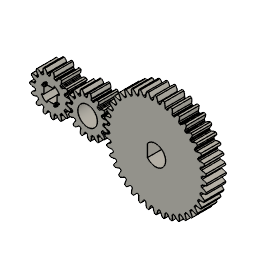
Dribbler Gears (Autodesk Fusion 360 design; units mm, degrees)
description: Spur Gear; Module: 1.5; Num Teeth: 18; Pressure Angle: 20.0; Backlash: 0.00 mm
part number: 2026-04-08-17-27-07-443
Autodesk Fusion 360 part; units mm, degrees
(part 1 of 6)
sketch "Base Circle" plane through (0, 0, 0) normal (0, 0, 1) x (1, 0, 0)
  circle A0 centre (0, 0) radius 9.4215
  circle A1 centre (0, 0) radius 2
extrude "Extrude12" add sketch "Base Circle" along normal blind 4 makes body 1
sketch "Gear Tooth" plane through (0, 0, 0) normal (0, 0, 1) x (1, 0, 0)
  spline S0 degree 5 poles (9.3831, -0.5088) (9.3863, -0.5089) (9.3927, -0.5089) (9.4023, -0.5088) (9.415, -0.5086) (9.431, -0.5081) (9.4469, -0.5073) (9.4629, -0.5063) (9.4789, -0.505) (9.4949, -0.5035) (9.5109, -0.5018) (9.5269, -0.4999) (9.5428, -0.4978) (9.5588, -0.4956) (9.5749, -0.4933) (9.5909, -0.4909) (9.6069, -0.4883) (9.6229, -0.4856) (9.6389, -0.4827) (9.6549, -0.4797) (9.6709, -0.4766) (9.6869, -0.4734) (9.7029, -0.4701) (9.7189, -0.4667) (9.7349, -0.4631) (9.7509, -0.4595) (9.7669, -0.4557) (9.7829, -0.4519) (9.7989, -0.4479) (9.8149, -0.4439) (9.8309, -0.4397) (9.8469, -0.4355) (9.8629, -0.4311) (9.8788, -0.4267) (9.8948, -0.4222) (9.9108, -0.4176) (9.9268, -0.4129) (9.9428, -0.4081) (9.9587, -0.4032) (9.9747, -0.3982) (9.9906, -0.3931) (10.0066, -0.388) (10.0225, -0.3828) (10.0385, -0.3775) (10.0544, -0.3721) (10.0704, -0.3666) (10.0863, -0.3611) (10.1022, -0.3554) (10.1181, -0.3497) (10.1341, -0.3439) (10.15, -0.338) (10.1659, -0.3321) (10.1818, -0.3261) (10.1977, -0.32) (10.2136, -0.3138) (10.2294, -0.3075) (10.2453, -0.3012) (10.2612, -0.2948) (10.277, -0.2883) (10.2929, -0.2818) (10.3087, -0.2752) (10.3246, -0.2685) (10.3404, -0.2617) (10.3562, -0.2549) (10.372, -0.248) (10.3878, -0.241) (10.4036, -0.2339) (10.4194, -0.2268) (10.4352, -0.2196) (10.451, -0.2124) (10.4668, -0.205) (10.4794, -0.1991) (10.4888, -0.1946) (10.4951, -0.1917) (10.4983, -0.1902) knots 0 0 0 0 0 0 0.01428571 0.02857143 0.04285714 0.05714286 0.07142857 0.08571429 0.1 0.11428571 0.12857143 0.14285714 0.15714286 0.17142857 0.18571429 0.2 0.21428571 0.22857143 0.24285714 0.25714286 0.27142857 0.28571429 0.3 0.31428571 0.32857143 0.34285714 0.35714286 0.37142857 0.38571429 0.4 0.41428571 0.42857143 0.44285714 0.45714286 0.47142857 0.48571429 0.5 0.51428571 0.52857143 0.54285714 0.55714286 0.57142857 0.58571429 0.6 0.61428571 0.62857143 0.64285714 0.65714286 0.67142857 0.68571429 0.7 0.71428571 0.72857143 0.74285714 0.75714286 0.77142857 0.78571429 0.8 0.81428571 0.82857143 0.84285714 0.85714286 0.87142857 0.88571429 0.9 0.91428571 0.92857143 0.94285714 0.95714286 0.97142857 0.98571429 1 1 1 1 1 1
  spline S1 degree 5 poles (9.3831, 0.5088) (9.3863, 0.5089) (9.3927, 0.5089) (9.4023, 0.5088) (9.415, 0.5086) (9.431, 0.5081) (9.4469, 0.5073) (9.4629, 0.5063) (9.4789, 0.505) (9.4949, 0.5035) (9.5109, 0.5018) (9.5269, 0.4999) (9.5428, 0.4978) (9.5588, 0.4956) (9.5749, 0.4933) (9.5909, 0.4909) (9.6069, 0.4883) (9.6229, 0.4856) (9.6389, 0.4827) (9.6549, 0.4797) (9.6709, 0.4766) (9.6869, 0.4734) (9.7029, 0.4701) (9.7189, 0.4667) (9.7349, 0.4631) (9.7509, 0.4595) (9.7669, 0.4557) (9.7829, 0.4519) (9.7989, 0.4479) (9.8149, 0.4439) (9.8309, 0.4397) (9.8469, 0.4355) (9.8629, 0.4311) (9.8788, 0.4267) (9.8948, 0.4222) (9.9108, 0.4176) (9.9268, 0.4129) (9.9428, 0.4081) (9.9587, 0.4032) (9.9747, 0.3982) (9.9906, 0.3931) (10.0066, 0.388) (10.0225, 0.3828) (10.0385, 0.3775) (10.0544, 0.3721) (10.0704, 0.3666) (10.0863, 0.3611) (10.1022, 0.3554) (10.1181, 0.3497) (10.1341, 0.3439) (10.15, 0.338) (10.1659, 0.3321) (10.1818, 0.3261) (10.1977, 0.32) (10.2136, 0.3138) (10.2294, 0.3075) (10.2453, 0.3012) (10.2612, 0.2948) (10.277, 0.2883) (10.2929, 0.2818) (10.3087, 0.2752) (10.3246, 0.2685) (10.3404, 0.2617) (10.3562, 0.2549) (10.372, 0.248) (10.3878, 0.241) (10.4036, 0.2339) (10.4194, 0.2268) (10.4352, 0.2196) (10.451, 0.2124) (10.4668, 0.205) (10.4794, 0.1991) (10.4888, 0.1946) (10.4951, 0.1917) (10.4983, 0.1902) knots 0 0 0 0 0 0 0.01428571 0.02857143 0.04285714 0.05714286 0.07142857 0.08571429 0.1 0.11428571 0.12857143 0.14285714 0.15714286 0.17142857 0.18571429 0.2 0.21428571 0.22857143 0.24285714 0.25714286 0.27142857 0.28571429 0.3 0.31428571 0.32857143 0.34285714 0.35714286 0.37142857 0.38571429 0.4 0.41428571 0.42857143 0.44285714 0.45714286 0.47142857 0.48571429 0.5 0.51428571 0.52857143 0.54285714 0.55714286 0.57142857 0.58571429 0.6 0.61428571 0.62857143 0.64285714 0.65714286 0.67142857 0.68571429 0.7 0.71428571 0.72857143 0.74285714 0.75714286 0.77142857 0.78571429 0.8 0.81428571 0.82857143 0.84285714 0.85714286 0.87142857 0.88571429 0.9 0.91428571 0.92857143 0.94285714 0.95714286 0.97142857 0.98571429 1 1 1 1 1 1
  arc A0 (10.4983, -0.1902) -> (10.4983, 0.1902) centre (0, 0) ccw
  line L0 (9.3831, 0.5088) -> (9.3831, -0.5088)
  point P0 (9.4622, -0.5063)
  point P1 (9.5415, -0.498)
  point P2 (9.621, -0.4858)
  point P3 (9.7007, -0.4705)
  point P4 (9.7804, -0.4525)
  point P5 (9.8602, -0.4318)
  point P6 (9.9401, -0.4089)
  point P7 (10.0199, -0.3836)
  point P8 (10.0998, -0.3563)
  point P9 (10.1796, -0.3269)
  point P10 (10.2594, -0.2955)
  point P11 (10.3391, -0.2622)
  point P12 (10.4187, -0.2271)
  point P13 (9.4622, 0.5063)
  point P14 (9.5415, 0.498)
  point P15 (9.621, 0.4858)
  point P16 (9.7007, 0.4705)
  point P17 (9.7804, 0.4525)
  point P18 (9.8602, 0.4318)
  point P19 (9.9401, 0.4089)
  point P20 (10.0199, 0.3836)
  point P21 (10.0998, 0.3563)
  point P22 (10.1796, 0.3269)
  point P23 (10.2594, 0.2955)
  point P24 (10.3391, 0.2622)
  point P25 (10.4187, 0.2271)
extrude "Extrude13" add sketch "Gear Tooth" along normal blind 4 bodies 1
fillet "Fillet6" radius 0.2 2 edges at (9.4078, 0.5087, 2) (9.4078, -0.5087, 2) on bodies 1
pattern_circular "C-Pattern6" count 40 over 360 about axis through (0, 0, 0) along (0, 0, 1) of "Extrude13", "Fillet6"
sketch "Diametrial Pitch Circle" plane through (0, 0, 0) normal (0, 0, 1) x (1, 0, 0)
  circle A0 centre (0, 0) radius 10 construction
sketch "Base Circle (1)" plane through (0, 0, 0) normal (0, 0, 1) x (1, 0, 0)
  circle A0 centre (0, 0) radius 3.1715
  circle A1 centre (0, 0) radius 2
extrude "Extrude14" add sketch "Base Circle (1)" along normal blind 4 separate body makes body 2
sketch "Gear Tooth (1)" plane through (0, 0, 0) normal (0, 0, 1) x (1, 0, 0)
  spline S0 degree 5 poles (3.4987, -0.4205) (3.5008, -0.4208) (3.505, -0.4212) (3.5113, -0.4217) (3.5197, -0.422) (3.5303, -0.4219) (3.5409, -0.4214) (3.5515, -0.4208) (3.5621, -0.42) (3.5728, -0.4191) (3.5834, -0.4181) (3.5941, -0.4171) (3.6048, -0.4159) (3.6155, -0.4145) (3.6262, -0.413) (3.6369, -0.4113) (3.6476, -0.4094) (3.6584, -0.4075) (3.6691, -0.4054) (3.6799, -0.4033) (3.6906, -0.401) (3.7013, -0.3987) (3.7121, -0.3962) (3.7229, -0.3936) (3.7336, -0.391) (3.7444, -0.3882) (3.7552, -0.3853) (3.7659, -0.3824) (3.7767, -0.3793) (3.7875, -0.3761) (3.7982, -0.3729) (3.809, -0.3696) (3.8198, -0.3661) (3.8305, -0.3626) (3.8413, -0.359) (3.8521, -0.3554) (3.8629, -0.3516) (3.8736, -0.3477) (3.8844, -0.3438) (3.8951, -0.3398) (3.9059, -0.3357) (3.9167, -0.3315) (3.9274, -0.3272) (3.9381, -0.3229) (3.9489, -0.3184) (3.9596, -0.3139) (3.9704, -0.3093) (3.9811, -0.3047) (3.9918, -0.2999) (4.0025, -0.2951) (4.0132, -0.2902) (4.0239, -0.2853) (4.0346, -0.2802) (4.0453, -0.2751) (4.056, -0.2699) (4.0667, -0.2646) (4.0774, -0.2593) (4.088, -0.2539) (4.0987, -0.2484) (4.1093, -0.2428) (4.12, -0.2372) (4.1306, -0.2315) (4.1412, -0.2257) (4.1518, -0.2199) (4.1624, -0.2139) (4.173, -0.2079) (4.1836, -0.2019) (4.1942, -0.1958) (4.2047, -0.1896) (4.2153, -0.1833) (4.2258, -0.177) (4.2342, -0.1718) (4.2405, -0.168) (4.2447, -0.1654) (4.2468, -0.1641) knots 0 0 0 0 0 0 0.01428571 0.02857143 0.04285714 0.05714286 0.07142857 0.08571429 0.1 0.11428571 0.12857143 0.14285714 0.15714286 0.17142857 0.18571429 0.2 0.21428571 0.22857143 0.24285714 0.25714286 0.27142857 0.28571429 0.3 0.31428571 0.32857143 0.34285714 0.35714286 0.37142857 0.38571429 0.4 0.41428571 0.42857143 0.44285714 0.45714286 0.47142857 0.48571429 0.5 0.51428571 0.52857143 0.54285714 0.55714286 0.57142857 0.58571429 0.6 0.61428571 0.62857143 0.64285714 0.65714286 0.67142857 0.68571429 0.7 0.71428571 0.72857143 0.74285714 0.75714286 0.77142857 0.78571429 0.8 0.81428571 0.82857143 0.84285714 0.85714286 0.87142857 0.88571429 0.9 0.91428571 0.92857143 0.94285714 0.95714286 0.97142857 0.98571429 1 1 1 1 1 1
  spline S1 degree 5 poles (3.4987, 0.4205) (3.5008, 0.4208) (3.505, 0.4212) (3.5113, 0.4217) (3.5197, 0.422) (3.5303, 0.4219) (3.5409, 0.4214) (3.5515, 0.4208) (3.5621, 0.42) (3.5728, 0.4191) (3.5834, 0.4181) (3.5941, 0.4171) (3.6048, 0.4159) (3.6155, 0.4145) (3.6262, 0.413) (3.6369, 0.4113) (3.6476, 0.4094) (3.6584, 0.4075) (3.6691, 0.4054) (3.6799, 0.4033) (3.6906, 0.401) (3.7013, 0.3987) (3.7121, 0.3962) (3.7229, 0.3936) (3.7336, 0.391) (3.7444, 0.3882) (3.7552, 0.3853) (3.7659, 0.3824) (3.7767, 0.3793) (3.7875, 0.3761) (3.7982, 0.3729) (3.809, 0.3696) (3.8198, 0.3661) (3.8305, 0.3626) (3.8413, 0.359) (3.8521, 0.3554) (3.8629, 0.3516) (3.8736, 0.3477) (3.8844, 0.3438) (3.8951, 0.3398) (3.9059, 0.3357) (3.9167, 0.3315) (3.9274, 0.3272) (3.9381, 0.3229) (3.9489, 0.3184) (3.9596, 0.3139) (3.9704, 0.3093) (3.9811, 0.3047) (3.9918, 0.2999) (4.0025, 0.2951) (4.0132, 0.2902) (4.0239, 0.2853) (4.0346, 0.2802) (4.0453, 0.2751) (4.056, 0.2699) (4.0667, 0.2646) (4.0774, 0.2593) (4.088, 0.2539) (4.0987, 0.2484) (4.1093, 0.2428) (4.12, 0.2372) (4.1306, 0.2315) (4.1412, 0.2257) (4.1518, 0.2199) (4.1624, 0.2139) (4.173, 0.2079) (4.1836, 0.2019) (4.1942, 0.1958) (4.2047, 0.1896) (4.2153, 0.1833) (4.2258, 0.177) (4.2342, 0.1718) (4.2405, 0.168) (4.2447, 0.1654) (4.2468, 0.1641) knots 0 0 0 0 0 0 0.01428571 0.02857143 0.04285714 0.05714286 0.07142857 0.08571429 0.1 0.11428571 0.12857143 0.14285714 0.15714286 0.17142857 0.18571429 0.2 0.21428571 0.22857143 0.24285714 0.25714286 0.27142857 0.28571429 0.3 0.31428571 0.32857143 0.34285714 0.35714286 0.37142857 0.38571429 0.4 0.41428571 0.42857143 0.44285714 0.45714286 0.47142857 0.48571429 0.5 0.51428571 0.52857143 0.54285714 0.55714286 0.57142857 0.58571429 0.6 0.61428571 0.62857143 0.64285714 0.65714286 0.67142857 0.68571429 0.7 0.71428571 0.72857143 0.74285714 0.75714286 0.77142857 0.78571429 0.8 0.81428571 0.82857143 0.84285714 0.85714286 0.87142857 0.88571429 0.9 0.91428571 0.92857143 0.94285714 0.95714286 0.97142857 0.98571429 1 1 1 1 1 1
  arc A0 (4.2468, -0.1641) -> (4.2468, 0.1641) centre (0, 0) ccw
  line L0 (3.1389, -0.3773) -> (3.4987, -0.4205)
  line L1 (3.1389, 0.3773) -> (3.4987, 0.4205)
  line L2 (3.1389, -0.3773) -> (3.1389, 0.3773)
  point P0 (3.5509, -0.4208)
  point P1 (3.6037, -0.416)
  point P2 (3.6568, -0.4077)
  point P3 (3.7102, -0.3966)
  point P4 (3.7638, -0.3829)
  point P5 (3.8175, -0.3669)
  point P6 (3.8713, -0.3486)
  point P7 (3.9251, -0.3281)
  point P8 (3.9789, -0.3056)
  point P9 (4.0327, -0.2811)
  point P10 (4.0865, -0.2546)
  point P11 (4.1401, -0.2263)
  point P12 (4.1935, -0.1961)
  point P13 (3.5509, 0.4208)
  point P14 (3.6037, 0.416)
  point P15 (3.6568, 0.4077)
  point P16 (3.7102, 0.3966)
  point P17 (3.7638, 0.3829)
  point P18 (3.8175, 0.3669)
  point P19 (3.8713, 0.3486)
  point P20 (3.9251, 0.3281)
  point P21 (3.9789, 0.3056)
  point P22 (4.0327, 0.2811)
  point P23 (4.0865, 0.2546)
  point P24 (4.1401, 0.2263)
  point P25 (4.1935, 0.1961)
extrude "Extrude15" add sketch "Gear Tooth (1)" along normal blind 4 bodies 2
fillet "Fillet7" radius 0.2 2 edges at (3.1488, -0.3785, 2) (3.1488, 0.3785, 2) on bodies 2
pattern_circular "C-Pattern7" count 15 over 360 about axis through (0, 0, 0) along (0, 0, 1) of "Extrude15", "Fillet7"
sketch "Diametrial Pitch Circle (1)" plane through (0, 0, 0) normal (0, 0, 1) x (1, 0, 0)
  circle A0 centre (0, 0) radius 3.75 construction
move_body "Move5" bodies 2 to x (1, 0, 0) y (0, 1, 0) z (0, 0, 1) at (-13.9, 0, 0)
move_body "Move6" bodies 2 to x (0.978148, -0.207912, 0) y (0.207912, 0.978148, 0) z (0, 0, 1) at (-0.3037, -2.89, 0)
sketch "Base Circle (2)" plane through (0, 0, 0) normal (0, 0, 1) x (1, 0, 0)
  circle A0 centre (0, 0) radius 3.1715
  circle A1 centre (0, 0) radius 2
extrude "Extrude16" add sketch "Base Circle (2)" along normal blind 4 separate body makes body 3
sketch "Gear Tooth (2)" plane through (0, 0, 0) normal (0, 0, 1) x (1, 0, 0)
  spline S0 degree 5 poles (3.4987, -0.4205) (3.5008, -0.4208) (3.505, -0.4212) (3.5113, -0.4217) (3.5197, -0.422) (3.5303, -0.4219) (3.5409, -0.4214) (3.5515, -0.4208) (3.5621, -0.42) (3.5728, -0.4191) (3.5834, -0.4181) (3.5941, -0.4171) (3.6048, -0.4159) (3.6155, -0.4145) (3.6262, -0.413) (3.6369, -0.4113) (3.6476, -0.4094) (3.6584, -0.4075) (3.6691, -0.4054) (3.6799, -0.4033) (3.6906, -0.401) (3.7013, -0.3987) (3.7121, -0.3962) (3.7229, -0.3936) (3.7336, -0.391) (3.7444, -0.3882) (3.7552, -0.3853) (3.7659, -0.3824) (3.7767, -0.3793) (3.7875, -0.3761) (3.7982, -0.3729) (3.809, -0.3696) (3.8198, -0.3661) (3.8305, -0.3626) (3.8413, -0.359) (3.8521, -0.3554) (3.8629, -0.3516) (3.8736, -0.3477) (3.8844, -0.3438) (3.8951, -0.3398) (3.9059, -0.3357) (3.9167, -0.3315) (3.9274, -0.3272) (3.9381, -0.3229) (3.9489, -0.3184) (3.9596, -0.3139) (3.9704, -0.3093) (3.9811, -0.3047) (3.9918, -0.2999) (4.0025, -0.2951) (4.0132, -0.2902) (4.0239, -0.2853) (4.0346, -0.2802) (4.0453, -0.2751) (4.056, -0.2699) (4.0667, -0.2646) (4.0774, -0.2593) (4.088, -0.2539) (4.0987, -0.2484) (4.1093, -0.2428) (4.12, -0.2372) (4.1306, -0.2315) (4.1412, -0.2257) (4.1518, -0.2199) (4.1624, -0.2139) (4.173, -0.2079) (4.1836, -0.2019) (4.1942, -0.1958) (4.2047, -0.1896) (4.2153, -0.1833) (4.2258, -0.177) (4.2342, -0.1718) (4.2405, -0.168) (4.2447, -0.1654) (4.2468, -0.1641) knots 0 0 0 0 0 0 0.01428571 0.02857143 0.04285714 0.05714286 0.07142857 0.08571429 0.1 0.11428571 0.12857143 0.14285714 0.15714286 0.17142857 0.18571429 0.2 0.21428571 0.22857143 0.24285714 0.25714286 0.27142857 0.28571429 0.3 0.31428571 0.32857143 0.34285714 0.35714286 0.37142857 0.38571429 0.4 0.41428571 0.42857143 0.44285714 0.45714286 0.47142857 0.48571429 0.5 0.51428571 0.52857143 0.54285714 0.55714286 0.57142857 0.58571429 0.6 0.61428571 0.62857143 0.64285714 0.65714286 0.67142857 0.68571429 0.7 0.71428571 0.72857143 0.74285714 0.75714286 0.77142857 0.78571429 0.8 0.81428571 0.82857143 0.84285714 0.85714286 0.87142857 0.88571429 0.9 0.91428571 0.92857143 0.94285714 0.95714286 0.97142857 0.98571429 1 1 1 1 1 1
  spline S1 degree 5 poles (3.4987, 0.4205) (3.5008, 0.4208) (3.505, 0.4212) (3.5113, 0.4217) (3.5197, 0.422) (3.5303, 0.4219) (3.5409, 0.4214) (3.5515, 0.4208) (3.5621, 0.42) (3.5728, 0.4191) (3.5834, 0.4181) (3.5941, 0.4171) (3.6048, 0.4159) (3.6155, 0.4145) (3.6262, 0.413) (3.6369, 0.4113) (3.6476, 0.4094) (3.6584, 0.4075) (3.6691, 0.4054) (3.6799, 0.4033) (3.6906, 0.401) (3.7013, 0.3987) (3.7121, 0.3962) (3.7229, 0.3936) (3.7336, 0.391) (3.7444, 0.3882) (3.7552, 0.3853) (3.7659, 0.3824) (3.7767, 0.3793) (3.7875, 0.3761) (3.7982, 0.3729) (3.809, 0.3696) (3.8198, 0.3661) (3.8305, 0.3626) (3.8413, 0.359) (3.8521, 0.3554) (3.8629, 0.3516) (3.8736, 0.3477) (3.8844, 0.3438) (3.8951, 0.3398) (3.9059, 0.3357) (3.9167, 0.3315) (3.9274, 0.3272) (3.9381, 0.3229) (3.9489, 0.3184) (3.9596, 0.3139) (3.9704, 0.3093) (3.9811, 0.3047) (3.9918, 0.2999) (4.0025, 0.2951) (4.0132, 0.2902) (4.0239, 0.2853) (4.0346, 0.2802) (4.0453, 0.2751) (4.056, 0.2699) (4.0667, 0.2646) (4.0774, 0.2593) (4.088, 0.2539) (4.0987, 0.2484) (4.1093, 0.2428) (4.12, 0.2372) (4.1306, 0.2315) (4.1412, 0.2257) (4.1518, 0.2199) (4.1624, 0.2139) (4.173, 0.2079) (4.1836, 0.2019) (4.1942, 0.1958) (4.2047, 0.1896) (4.2153, 0.1833) (4.2258, 0.177) (4.2342, 0.1718) (4.2405, 0.168) (4.2447, 0.1654) (4.2468, 0.1641) knots 0 0 0 0 0 0 0.01428571 0.02857143 0.04285714 0.05714286 0.07142857 0.08571429 0.1 0.11428571 0.12857143 0.14285714 0.15714286 0.17142857 0.18571429 0.2 0.21428571 0.22857143 0.24285714 0.25714286 0.27142857 0.28571429 0.3 0.31428571 0.32857143 0.34285714 0.35714286 0.37142857 0.38571429 0.4 0.41428571 0.42857143 0.44285714 0.45714286 0.47142857 0.48571429 0.5 0.51428571 0.52857143 0.54285714 0.55714286 0.57142857 0.58571429 0.6 0.61428571 0.62857143 0.64285714 0.65714286 0.67142857 0.68571429 0.7 0.71428571 0.72857143 0.74285714 0.75714286 0.77142857 0.78571429 0.8 0.81428571 0.82857143 0.84285714 0.85714286 0.87142857 0.88571429 0.9 0.91428571 0.92857143 0.94285714 0.95714286 0.97142857 0.98571429 1 1 1 1 1 1
  arc A0 (4.2468, -0.1641) -> (4.2468, 0.1641) centre (0, 0) ccw
  line L0 (3.1389, -0.3773) -> (3.4987, -0.4205)
  line L1 (3.1389, 0.3773) -> (3.4987, 0.4205)
  line L2 (3.1389, -0.3773) -> (3.1389, 0.3773)
  point P0 (3.5509, -0.4208)
  point P1 (3.6037, -0.416)
  point P2 (3.6568, -0.4077)
  point P3 (3.7102, -0.3966)
  point P4 (3.7638, -0.3829)
  point P5 (3.8175, -0.3669)
  point P6 (3.8713, -0.3486)
  point P7 (3.9251, -0.3281)
  point P8 (3.9789, -0.3056)
  point P9 (4.0327, -0.2811)
  point P10 (4.0865, -0.2546)
  point P11 (4.1401, -0.2263)
  point P12 (4.1935, -0.1961)
  point P13 (3.5509, 0.4208)
  point P14 (3.6037, 0.416)
  point P15 (3.6568, 0.4077)
  point P16 (3.7102, 0.3966)
  point P17 (3.7638, 0.3829)
  point P18 (3.8175, 0.3669)
  point P19 (3.8713, 0.3486)
  point P20 (3.9251, 0.3281)
  point P21 (3.9789, 0.3056)
  point P22 (4.0327, 0.2811)
  point P23 (4.0865, 0.2546)
  point P24 (4.1401, 0.2263)
  point P25 (4.1935, 0.1961)
extrude "Extrude17" add sketch "Gear Tooth (2)" along normal blind 4 bodies 3
fillet "Fillet8" radius 0.2 2 edges at (3.1488, -0.3785, 2) (3.1488, 0.3785, 2) on bodies 3
pattern_circular "C-Pattern8" count 15 over 360 about axis through (0, 0, 0) along (0, 0, 1) of "Extrude17", "Fillet8"
sketch "Diametrial Pitch Circle (2)" plane through (0, 0, 0) normal (0, 0, 1) x (1, 0, 0)
  circle A0 centre (0, 0) radius 3.75 construction
move_body "Move7" bodies 3 to x (1, 0, 0) y (0, 1, 0) z (0, 0, 1) at (-21.5, 0, 0)
move_body "Move8" bodies 3 to x (0.978148, -0.207912, 0) y (0.207912, 0.978148, 0) z (0, 0, 1) at (-0.4698, -4.4701, 0)
sketch "Sketch26" plane through (0, 0, 4) normal (0, 0, 1) x (1, 0, 0)
  arc A0 (-18.6433, -1.3776) -> (-18.5647, -1.2011) centre (-21.5, 0) ccw
  arc A1 (-18.315, -1.0876) -> (-18.5647, -1.2011) centre (-18.3796, -1.2769) ccw
  line L0 (-18.315, -1.0876) -> (-18.1652, -1.1388)
  spline S0 degree 5 poles (-18.1652, -1.1388) (-18.1632, -1.1394) (-18.1592, -1.1407) (-18.1531, -1.1425) (-18.145, -1.1446) (-18.1346, -1.1467) (-18.1241, -1.1484) (-18.1136, -1.15) (-18.103, -1.1514) (-18.0924, -1.1528) (-18.0818, -1.1541) (-18.0711, -1.1552) (-18.0604, -1.1563) (-18.0497, -1.1572) (-18.0389, -1.1579) (-18.0281, -1.1584) (-18.0172, -1.1589) (-18.0063, -1.1592) (-17.9954, -1.1594) (-17.9844, -1.1595) (-17.9734, -1.1596) (-17.9624, -1.1595) (-17.9514, -1.1593) (-17.9403, -1.1591) (-17.9293, -1.1587) (-17.9181, -1.1582) (-17.907, -1.1576) (-17.8959, -1.157) (-17.8847, -1.1562) (-17.8735, -1.1554) (-17.8623, -1.1544) (-17.8511, -1.1534) (-17.8398, -1.1523) (-17.8286, -1.1511) (-17.8173, -1.1498) (-17.806, -1.1485) (-17.7947, -1.147) (-17.7833, -1.1455) (-17.772, -1.1439) (-17.7606, -1.1422) (-17.7492, -1.1404) (-17.7379, -1.1385) (-17.7265, -1.1366) (-17.715, -1.1346) (-17.7036, -1.1325) (-17.6922, -1.1303) (-17.6807, -1.1281) (-17.6692, -1.1257) (-17.6578, -1.1233) (-17.6463, -1.1208) (-17.6348, -1.1183) (-17.6233, -1.1156) (-17.6118, -1.1129) (-17.6003, -1.1102) (-17.5887, -1.1073) (-17.5772, -1.1044) (-17.5656, -1.1013) (-17.5541, -1.0983) (-17.5425, -1.0951) (-17.5309, -1.0919) (-17.5194, -1.0886) (-17.5078, -1.0852) (-17.4962, -1.0818) (-17.4846, -1.0783) (-17.473, -1.0747) (-17.4614, -1.071) (-17.4498, -1.0673) (-17.4382, -1.0635) (-17.4266, -1.0596) (-17.415, -1.0557) (-17.4033, -1.0517) (-17.394, -1.0484) (-17.3871, -1.0459) (-17.3824, -1.0443) (-17.3801, -1.0434) knots 0 0 0 0 0 0 0.01428571 0.02857143 0.04285714 0.05714286 0.07142857 0.08571429 0.1 0.11428571 0.12857143 0.14285714 0.15714286 0.17142857 0.18571429 0.2 0.21428571 0.22857143 0.24285714 0.25714286 0.27142857 0.28571429 0.3 0.31428571 0.32857143 0.34285714 0.35714286 0.37142857 0.38571429 0.4 0.41428571 0.42857143 0.44285714 0.45714286 0.47142857 0.48571429 0.5 0.51428571 0.52857143 0.54285714 0.55714286 0.57142857 0.58571429 0.6 0.61428571 0.62857143 0.64285714 0.65714286 0.67142857 0.68571429 0.7 0.71428571 0.72857143 0.74285714 0.75714286 0.77142857 0.78571429 0.8 0.81428571 0.82857143 0.84285714 0.85714286 0.87142857 0.88571429 0.9 0.91428571 0.92857143 0.94285714 0.95714286 0.97142857 0.98571429 1 1 1 1 1 1
  arc A2 (-17.3801, -1.0434) -> (-17.3119, -0.7225) centre (-21.5, 0) ccw
  spline S1 degree 5 poles (-17.3119, -0.7225) (-17.3136, -0.7208) (-17.3172, -0.7174) (-17.3226, -0.7123) (-17.3298, -0.7055) (-17.3387, -0.6971) (-17.3478, -0.6888) (-17.3568, -0.6805) (-17.3659, -0.6723) (-17.3749, -0.6642) (-17.3841, -0.6562) (-17.3932, -0.6482) (-17.4024, -0.6402) (-17.4115, -0.6324) (-17.4207, -0.6246) (-17.43, -0.6169) (-17.4392, -0.6092) (-17.4485, -0.6016) (-17.4578, -0.5941) (-17.4671, -0.5867) (-17.4765, -0.5793) (-17.4859, -0.572) (-17.4953, -0.5648) (-17.5047, -0.5576) (-17.5141, -0.5505) (-17.5236, -0.5435) (-17.5331, -0.5366) (-17.5426, -0.5297) (-17.5521, -0.5229) (-17.5616, -0.5162) (-17.5712, -0.5095) (-17.5808, -0.503) (-17.5904, -0.4965) (-17.6, -0.4901) (-17.6097, -0.4838) (-17.6193, -0.4775) (-17.629, -0.4713) (-17.6387, -0.4652) (-17.6485, -0.4592) (-17.6582, -0.4533) (-17.668, -0.4475) (-17.6778, -0.4417) (-17.6876, -0.436) (-17.6974, -0.4304) (-17.7072, -0.4249) (-17.7171, -0.4195) (-17.727, -0.4142) (-17.7369, -0.409) (-17.7468, -0.4038) (-17.7567, -0.3988) (-17.7667, -0.3938) (-17.7766, -0.389) (-17.7866, -0.3842) (-17.7966, -0.3796) (-17.8067, -0.3751) (-17.8167, -0.3706) (-17.8268, -0.3663) (-17.8369, -0.362) (-17.8469, -0.3579) (-17.857, -0.3539) (-17.8672, -0.35) (-17.8773, -0.3463) (-17.8875, -0.3427) (-17.8977, -0.3393) (-17.9079, -0.336) (-17.9182, -0.3329) (-17.9284, -0.3298) (-17.9386, -0.3268) (-17.9489, -0.324) (-17.9592, -0.3213) (-17.9695, -0.319) (-17.9778, -0.3175) (-17.9841, -0.3167) (-17.9883, -0.3163) (-17.9904, -0.3161) knots -1 -1 -1 -1 -1 -1 -0.98571429 -0.97142857 -0.95714286 -0.94285714 -0.92857143 -0.91428571 -0.9 -0.88571429 -0.87142857 -0.85714286 -0.84285714 -0.82857143 -0.81428571 -0.8 -0.78571429 -0.77142857 -0.75714286 -0.74285714 -0.72857143 -0.71428571 -0.7 -0.68571429 -0.67142857 -0.65714286 -0.64285714 -0.62857143 -0.61428571 -0.6 -0.58571429 -0.57142857 -0.55714286 -0.54285714 -0.52857143 -0.51428571 -0.5 -0.48571429 -0.47142857 -0.45714286 -0.44285714 -0.42857143 -0.41428571 -0.4 -0.38571429 -0.37142857 -0.35714286 -0.34285714 -0.32857143 -0.31428571 -0.3 -0.28571429 -0.27142857 -0.25714286 -0.24285714 -0.22857143 -0.21428571 -0.2 -0.18571429 -0.17142857 -0.15714286 -0.14285714 -0.12857143 -0.11428571 -0.1 -0.08571429 -0.07142857 -0.05714286 -0.04285714 -0.02857143 -0.01428571 0 0 0 0 0 0
  line L1 (-17.9904, -0.3161) -> (-18.148, -0.3019)
  arc A3 (-18.33, -0.0966) -> (-18.148, -0.3019) centre (-18.1301, -0.1027) ccw
  arc A4 (-18.33, -0.0966) -> (-18.33, 0.0966) centre (-21.5, 0) ccw
  arc A5 (-18.148, 0.3019) -> (-18.33, 0.0966) centre (-18.1301, 0.1027) ccw
  line L2 (-18.148, 0.3019) -> (-17.9904, 0.3161)
  spline S2 degree 5 poles (-17.9904, 0.3161) (-17.9883, 0.3163) (-17.9841, 0.3167) (-17.9778, 0.3175) (-17.9695, 0.319) (-17.9592, 0.3213) (-17.9489, 0.324) (-17.9386, 0.3268) (-17.9284, 0.3298) (-17.9182, 0.3329) (-17.9079, 0.336) (-17.8977, 0.3393) (-17.8875, 0.3427) (-17.8773, 0.3463) (-17.8672, 0.35) (-17.857, 0.3539) (-17.8469, 0.3579) (-17.8369, 0.362) (-17.8268, 0.3663) (-17.8167, 0.3706) (-17.8067, 0.3751) (-17.7966, 0.3796) (-17.7866, 0.3842) (-17.7766, 0.389) (-17.7667, 0.3938) (-17.7567, 0.3988) (-17.7468, 0.4038) (-17.7369, 0.409) (-17.727, 0.4142) (-17.7171, 0.4195) (-17.7072, 0.4249) (-17.6974, 0.4304) (-17.6876, 0.436) (-17.6778, 0.4417) (-17.668, 0.4475) (-17.6582, 0.4533) (-17.6485, 0.4592) (-17.6387, 0.4652) (-17.629, 0.4713) (-17.6193, 0.4775) (-17.6097, 0.4838) (-17.6, 0.4901) (-17.5904, 0.4965) (-17.5808, 0.503) (-17.5712, 0.5095) (-17.5616, 0.5162) (-17.5521, 0.5229) (-17.5426, 0.5297) (-17.5331, 0.5366) (-17.5236, 0.5435) (-17.5141, 0.5505) (-17.5047, 0.5576) (-17.4953, 0.5648) (-17.4859, 0.572) (-17.4765, 0.5793) (-17.4671, 0.5867) (-17.4578, 0.5941) (-17.4485, 0.6016) (-17.4392, 0.6092) (-17.43, 0.6169) (-17.4207, 0.6246) (-17.4115, 0.6324) (-17.4024, 0.6402) (-17.3932, 0.6482) (-17.3841, 0.6562) (-17.3749, 0.6642) (-17.3659, 0.6723) (-17.3568, 0.6805) (-17.3478, 0.6888) (-17.3387, 0.6971) (-17.3298, 0.7055) (-17.3226, 0.7123) (-17.3172, 0.7174) (-17.3136, 0.7208) (-17.3119, 0.7225) knots 0 0 0 0 0 0 0.01428571 0.02857143 0.04285714 0.05714286 0.07142857 0.08571429 0.1 0.11428571 0.12857143 0.14285714 0.15714286 0.17142857 0.18571429 0.2 0.21428571 0.22857143 0.24285714 0.25714286 0.27142857 0.28571429 0.3 0.31428571 0.32857143 0.34285714 0.35714286 0.37142857 0.38571429 0.4 0.41428571 0.42857143 0.44285714 0.45714286 0.47142857 0.48571429 0.5 0.51428571 0.52857143 0.54285714 0.55714286 0.57142857 0.58571429 0.6 0.61428571 0.62857143 0.64285714 0.65714286 0.67142857 0.68571429 0.7 0.71428571 0.72857143 0.74285714 0.75714286 0.77142857 0.78571429 0.8 0.81428571 0.82857143 0.84285714 0.85714286 0.87142857 0.88571429 0.9 0.91428571 0.92857143 0.94285714 0.95714286 0.97142857 0.98571429 1 1 1 1 1 1
  arc A6 (-17.3119, 0.7225) -> (-17.3801, 1.0434) centre (-21.5, 0) ccw
  spline S3 degree 5 poles (-17.3801, 1.0434) (-17.3824, 1.0443) (-17.3871, 1.0459) (-17.394, 1.0484) (-17.4033, 1.0517) (-17.415, 1.0557) (-17.4266, 1.0596) (-17.4382, 1.0635) (-17.4498, 1.0673) (-17.4614, 1.071) (-17.473, 1.0747) (-17.4846, 1.0783) (-17.4962, 1.0818) (-17.5078, 1.0852) (-17.5194, 1.0886) (-17.5309, 1.0919) (-17.5425, 1.0951) (-17.5541, 1.0983) (-17.5656, 1.1013) (-17.5772, 1.1044) (-17.5887, 1.1073) (-17.6003, 1.1102) (-17.6118, 1.1129) (-17.6233, 1.1156) (-17.6348, 1.1183) (-17.6463, 1.1208) (-17.6578, 1.1233) (-17.6692, 1.1257) (-17.6807, 1.1281) (-17.6922, 1.1303) (-17.7036, 1.1325) (-17.715, 1.1346) (-17.7265, 1.1366) (-17.7379, 1.1385) (-17.7492, 1.1404) (-17.7606, 1.1422) (-17.772, 1.1439) (-17.7833, 1.1455) (-17.7947, 1.147) (-17.806, 1.1485) (-17.8173, 1.1498) (-17.8286, 1.1511) (-17.8398, 1.1523) (-17.8511, 1.1534) (-17.8623, 1.1544) (-17.8735, 1.1554) (-17.8847, 1.1562) (-17.8959, 1.157) (-17.907, 1.1576) (-17.9181, 1.1582) (-17.9293, 1.1587) (-17.9403, 1.1591) (-17.9514, 1.1593) (-17.9624, 1.1595) (-17.9734, 1.1596) (-17.9844, 1.1595) (-17.9954, 1.1594) (-18.0063, 1.1592) (-18.0172, 1.1589) (-18.0281, 1.1584) (-18.0389, 1.1579) (-18.0497, 1.1572) (-18.0604, 1.1563) (-18.0711, 1.1552) (-18.0818, 1.1541) (-18.0924, 1.1528) (-18.103, 1.1514) (-18.1136, 1.15) (-18.1241, 1.1484) (-18.1346, 1.1467) (-18.145, 1.1446) (-18.1531, 1.1425) (-18.1592, 1.1407) (-18.1632, 1.1394) (-18.1652, 1.1388) knots -1 -1 -1 -1 -1 -1 -0.98571429 -0.97142857 -0.95714286 -0.94285714 -0.92857143 -0.91428571 -0.9 -0.88571429 -0.87142857 -0.85714286 -0.84285714 -0.82857143 -0.81428571 -0.8 -0.78571429 -0.77142857 -0.75714286 -0.74285714 -0.72857143 -0.71428571 -0.7 -0.68571429 -0.67142857 -0.65714286 -0.64285714 -0.62857143 -0.61428571 -0.6 -0.58571429 -0.57142857 -0.55714286 -0.54285714 -0.52857143 -0.51428571 -0.5 -0.48571429 -0.47142857 -0.45714286 -0.44285714 -0.42857143 -0.41428571 -0.4 -0.38571429 -0.37142857 -0.35714286 -0.34285714 -0.32857143 -0.31428571 -0.3 -0.28571429 -0.27142857 -0.25714286 -0.24285714 -0.22857143 -0.21428571 -0.2 -0.18571429 -0.17142857 -0.15714286 -0.14285714 -0.12857143 -0.11428571 -0.1 -0.08571429 -0.07142857 -0.05714286 -0.04285714 -0.02857143 -0.01428571 0 0 0 0 0 0
  line L3 (-18.1652, 1.1388) -> (-18.315, 1.0876)
  arc A7 (-18.5647, 1.2011) -> (-18.315, 1.0876) centre (-18.3796, 1.2769) ccw
  arc A8 (-18.5647, 1.2011) -> (-18.6433, 1.3776) centre (-21.5, 0) ccw
  arc A9 (-18.5606, 1.6392) -> (-18.6433, 1.3776) centre (-18.4632, 1.4645) ccw
  line L4 (-18.5606, 1.6392) -> (-18.4223, 1.7162)
  spline S4 degree 5 poles (-18.4223, 1.7162) (-18.4205, 1.7173) (-18.4168, 1.7194) (-18.4115, 1.7227) (-18.4045, 1.7274) (-18.396, 1.7337) (-18.3877, 1.7403) (-18.3795, 1.7471) (-18.3713, 1.754) (-18.3632, 1.761) (-18.3552, 1.768) (-18.3471, 1.7751) (-18.3392, 1.7824) (-18.3314, 1.7898) (-18.3236, 1.7973) (-18.3159, 1.805) (-18.3083, 1.8128) (-18.3008, 1.8207) (-18.2933, 1.8287) (-18.2859, 1.8367) (-18.2785, 1.8449) (-18.2712, 1.8531) (-18.264, 1.8614) (-18.2568, 1.8698) (-18.2496, 1.8783) (-18.2425, 1.8868) (-18.2355, 1.8955) (-18.2286, 1.9042) (-18.2216, 1.913) (-18.2148, 1.9219) (-18.208, 1.9309) (-18.2012, 1.9399) (-18.1945, 1.949) (-18.1879, 1.9582) (-18.1813, 1.9674) (-18.1747, 1.9767) (-18.1682, 1.9861) (-18.1618, 1.9955) (-18.1554, 2.0051) (-18.1491, 2.0146) (-18.1428, 2.0243) (-18.1365, 2.034) (-18.1303, 2.0438) (-18.1242, 2.0536) (-18.1181, 2.0635) (-18.1121, 2.0734) (-18.1061, 2.0835) (-18.1001, 2.0935) (-18.0943, 2.1037) (-18.0884, 2.1139) (-18.0826, 2.1241) (-18.0769, 2.1344) (-18.0712, 2.1448) (-18.0656, 2.1552) (-18.06, 2.1657) (-18.0544, 2.1763) (-18.0489, 2.1869) (-18.0435, 2.1975) (-18.0381, 2.2082) (-18.0328, 2.219) (-18.0275, 2.2298) (-18.0222, 2.2406) (-18.017, 2.2516) (-18.0119, 2.2625) (-18.0068, 2.2735) (-18.0017, 2.2846) (-17.9967, 2.2957) (-17.9918, 2.3069) (-17.9869, 2.3181) (-17.982, 2.3294) (-17.9772, 2.3407) (-17.9734, 2.3498) (-17.9706, 2.3566) (-17.9687, 2.3612) (-17.9678, 2.3635) knots 0 0 0 0 0 0 0.01428571 0.02857143 0.04285714 0.05714286 0.07142857 0.08571429 0.1 0.11428571 0.12857143 0.14285714 0.15714286 0.17142857 0.18571429 0.2 0.21428571 0.22857143 0.24285714 0.25714286 0.27142857 0.28571429 0.3 0.31428571 0.32857143 0.34285714 0.35714286 0.37142857 0.38571429 0.4 0.41428571 0.42857143 0.44285714 0.45714286 0.47142857 0.48571429 0.5 0.51428571 0.52857143 0.54285714 0.55714286 0.57142857 0.58571429 0.6 0.61428571 0.62857143 0.64285714 0.65714286 0.67142857 0.68571429 0.7 0.71428571 0.72857143 0.74285714 0.75714286 0.77142857 0.78571429 0.8 0.81428571 0.82857143 0.84285714 0.85714286 0.87142857 0.88571429 0.9 0.91428571 0.92857143 0.94285714 0.95714286 0.97142857 0.98571429 1 1 1 1 1 1
  arc A10 (-17.9678, 2.3635) -> (-18.1607, 2.629) centre (-21.5, 0) ccw
  spline S5 degree 5 poles (-18.1607, 2.629) (-18.1631, 2.6288) (-18.1681, 2.6284) (-18.1754, 2.6278) (-18.1853, 2.627) (-18.1975, 2.626) (-18.2097, 2.6248) (-18.2219, 2.6236) (-18.2341, 2.6224) (-18.2462, 2.6211) (-18.2583, 2.6197) (-18.2703, 2.6182) (-18.2823, 2.6167) (-18.2943, 2.6152) (-18.3063, 2.6135) (-18.3182, 2.6118) (-18.3301, 2.6101) (-18.3419, 2.6083) (-18.3537, 2.6064) (-18.3655, 2.6044) (-18.3772, 2.6024) (-18.3889, 2.6003) (-18.4006, 2.5982) (-18.4122, 2.596) (-18.4238, 2.5937) (-18.4353, 2.5914) (-18.4468, 2.589) (-18.4583, 2.5865) (-18.4697, 2.584) (-18.4811, 2.5814) (-18.4924, 2.5787) (-18.5037, 2.576) (-18.515, 2.5732) (-18.5262, 2.5703) (-18.5374, 2.5674) (-18.5485, 2.5644) (-18.5595, 2.5613) (-18.5706, 2.5582) (-18.5815, 2.555) (-18.5925, 2.5517) (-18.6033, 2.5483) (-18.6142, 2.5449) (-18.625, 2.5414) (-18.6357, 2.5379) (-18.6463, 2.5342) (-18.657, 2.5305) (-18.6675, 2.5267) (-18.678, 2.5229) (-18.6885, 2.519) (-18.6989, 2.515) (-18.7092, 2.5109) (-18.7195, 2.5067) (-18.7297, 2.5025) (-18.7399, 2.4981) (-18.75, 2.4937) (-18.76, 2.4892) (-18.7699, 2.4846) (-18.7798, 2.48) (-18.7897, 2.4753) (-18.7994, 2.4705) (-18.8091, 2.4655) (-18.8186, 2.4605) (-18.8281, 2.4553) (-18.8375, 2.45) (-18.8467, 2.4446) (-18.8559, 2.4391) (-18.865, 2.4335) (-18.8741, 2.4279) (-18.8831, 2.4222) (-18.8919, 2.4164) (-18.9006, 2.4102) (-18.9072, 2.405) (-18.912, 2.4009) (-18.9152, 2.3981) (-18.9167, 2.3967) knots -1 -1 -1 -1 -1 -1 -0.98571429 -0.97142857 -0.95714286 -0.94285714 -0.92857143 -0.91428571 -0.9 -0.88571429 -0.87142857 -0.85714286 -0.84285714 -0.82857143 -0.81428571 -0.8 -0.78571429 -0.77142857 -0.75714286 -0.74285714 -0.72857143 -0.71428571 -0.7 -0.68571429 -0.67142857 -0.65714286 -0.64285714 -0.62857143 -0.61428571 -0.6 -0.58571429 -0.57142857 -0.55714286 -0.54285714 -0.52857143 -0.51428571 -0.5 -0.48571429 -0.47142857 -0.45714286 -0.44285714 -0.42857143 -0.41428571 -0.4 -0.38571429 -0.37142857 -0.35714286 -0.34285714 -0.32857143 -0.31428571 -0.3 -0.28571429 -0.27142857 -0.25714286 -0.24285714 -0.22857143 -0.21428571 -0.2 -0.18571429 -0.17142857 -0.15714286 -0.14285714 -0.12857143 -0.11428571 -0.1 -0.08571429 -0.07142857 -0.05714286 -0.04285714 -0.02857143 -0.01428571 0 0 0 0 0 0
  line L5 (-18.9167, 2.3967) -> (-19.0327, 2.289)
  arc A11 (-19.3071, 2.2912) -> (-19.0327, 2.289) centre (-19.1688, 2.4356) ccw
  arc A12 (-19.3071, 2.2912) -> (-19.4506, 2.4204) centre (-21.5, 0) ccw
  arc A13 (-19.4814, 2.693) -> (-19.4506, 2.4204) centre (-19.3214, 2.5731) ccw
  line L6 (-19.4814, 2.693) -> (-19.3865, 2.8197)
  spline S6 degree 5 poles (-19.3865, 2.8197) (-19.3852, 2.8214) (-19.3827, 2.8248) (-19.3792, 2.83) (-19.3747, 2.8371) (-19.3695, 2.8463) (-19.3646, 2.8558) (-19.3599, 2.8653) (-19.3552, 2.8749) (-19.3507, 2.8846) (-19.3462, 2.8943) (-19.3417, 2.9041) (-19.3374, 2.9139) (-19.3333, 2.9239) (-19.3293, 2.9339) (-19.3254, 2.944) (-19.3216, 2.9542) (-19.3179, 2.9645) (-19.3143, 2.9748) (-19.3108, 2.9852) (-19.3074, 2.9956) (-19.3041, 3.0061) (-19.3008, 3.0167) (-19.2977, 3.0273) (-19.2946, 3.0379) (-19.2916, 3.0486) (-19.2887, 3.0594) (-19.2859, 3.0702) (-19.2832, 3.0811) (-19.2805, 3.092) (-19.2779, 3.1029) (-19.2754, 3.1139) (-19.273, 3.1249) (-19.2707, 3.136) (-19.2684, 3.1472) (-19.2662, 3.1583) (-19.2641, 3.1695) (-19.2621, 3.1808) (-19.2601, 3.1921) (-19.2582, 3.2034) (-19.2564, 3.2148) (-19.2546, 3.2262) (-19.2529, 3.2376) (-19.2513, 3.2491) (-19.2498, 3.2606) (-19.2483, 3.2722) (-19.2469, 3.2838) (-19.2456, 3.2954) (-19.2443, 3.307) (-19.2432, 3.3187) (-19.242, 3.3305) (-19.241, 3.3422) (-19.24, 3.354) (-19.2391, 3.3658) (-19.2383, 3.3777) (-19.2375, 3.3896) (-19.2368, 3.4015) (-19.2361, 3.4134) (-19.2356, 3.4254) (-19.235, 3.4374) (-19.2346, 3.4494) (-19.2342, 3.4615) (-19.2339, 3.4735) (-19.2337, 3.4857) (-19.2335, 3.4978) (-19.2334, 3.51) (-19.2334, 3.5222) (-19.2334, 3.5344) (-19.2335, 3.5466) (-19.2336, 3.5589) (-19.2339, 3.5712) (-19.2341, 3.581) (-19.2343, 3.5884) (-19.2344, 3.5934) (-19.2345, 3.5958) knots 0 0 0 0 0 0 0.01428571 0.02857143 0.04285714 0.05714286 0.07142857 0.08571429 0.1 0.11428571 0.12857143 0.14285714 0.15714286 0.17142857 0.18571429 0.2 0.21428571 0.22857143 0.24285714 0.25714286 0.27142857 0.28571429 0.3 0.31428571 0.32857143 0.34285714 0.35714286 0.37142857 0.38571429 0.4 0.41428571 0.42857143 0.44285714 0.45714286 0.47142857 0.48571429 0.5 0.51428571 0.52857143 0.54285714 0.55714286 0.57142857 0.58571429 0.6 0.61428571 0.62857143 0.64285714 0.65714286 0.67142857 0.68571429 0.7 0.71428571 0.72857143 0.74285714 0.75714286 0.77142857 0.78571429 0.8 0.81428571 0.82857143 0.84285714 0.85714286 0.87142857 0.88571429 0.9 0.91428571 0.92857143 0.94285714 0.95714286 0.97142857 0.98571429 1 1 1 1 1 1
  arc A14 (-19.2345, 3.5958) -> (-19.5187, 3.7599) centre (-21.5, 0) ccw
  spline S7 degree 5 poles (-19.5187, 3.7599) (-19.5208, 3.7587) (-19.5252, 3.7564) (-19.5317, 3.7529) (-19.5403, 3.7481) (-19.5511, 3.7422) (-19.5618, 3.7362) (-19.5724, 3.7301) (-19.583, 3.724) (-19.5936, 3.7179) (-19.6041, 3.7117) (-19.6145, 3.7055) (-19.6249, 3.6993) (-19.6352, 3.6929) (-19.6454, 3.6866) (-19.6556, 3.6802) (-19.6658, 3.6738) (-19.6758, 3.6673) (-19.6859, 3.6607) (-19.6958, 3.6542) (-19.7057, 3.6476) (-19.7156, 3.6409) (-19.7253, 3.6342) (-19.7351, 3.6275) (-19.7447, 3.6207) (-19.7543, 3.6139) (-19.7638, 3.607) (-19.7733, 3.6001) (-19.7827, 3.5931) (-19.792, 3.5861) (-19.8013, 3.5791) (-19.8105, 3.572) (-19.8197, 3.5648) (-19.8287, 3.5577) (-19.8377, 3.5504) (-19.8467, 3.5432) (-19.8555, 3.5359) (-19.8643, 3.5285) (-19.8731, 3.5211) (-19.8817, 3.5137) (-19.8903, 3.5062) (-19.8988, 3.4987) (-19.9072, 3.4911) (-19.9156, 3.4835) (-19.9238, 3.4758) (-19.932, 3.4681) (-19.9401, 3.4604) (-19.9482, 3.4526) (-19.9561, 3.4447) (-19.964, 3.4368) (-19.9718, 3.4289) (-19.9795, 3.4209) (-19.9871, 3.4129) (-19.9946, 3.4048) (-20.002, 3.3967) (-20.0093, 3.3885) (-20.0165, 3.3802) (-20.0237, 3.372) (-20.0308, 3.3637) (-20.0377, 3.3553) (-20.0445, 3.3469) (-20.0512, 3.3384) (-20.0578, 3.3298) (-20.0641, 3.3211) (-20.0704, 3.3124) (-20.0766, 3.3037) (-20.0826, 3.2949) (-20.0887, 3.2861) (-20.0945, 3.2772) (-20.1002, 3.2682) (-20.1056, 3.2591) (-20.1096, 3.2517) (-20.1123, 3.246) (-20.114, 3.2421) (-20.1149, 3.2402) knots -1 -1 -1 -1 -1 -1 -0.98571429 -0.97142857 -0.95714286 -0.94285714 -0.92857143 -0.91428571 -0.9 -0.88571429 -0.87142857 -0.85714286 -0.84285714 -0.82857143 -0.81428571 -0.8 -0.78571429 -0.77142857 -0.75714286 -0.74285714 -0.72857143 -0.71428571 -0.7 -0.68571429 -0.67142857 -0.65714286 -0.64285714 -0.62857143 -0.61428571 -0.6 -0.58571429 -0.57142857 -0.55714286 -0.54285714 -0.52857143 -0.51428571 -0.5 -0.48571429 -0.47142857 -0.45714286 -0.44285714 -0.42857143 -0.41428571 -0.4 -0.38571429 -0.37142857 -0.35714286 -0.34285714 -0.32857143 -0.31428571 -0.3 -0.28571429 -0.27142857 -0.25714286 -0.24285714 -0.22857143 -0.21428571 -0.2 -0.18571429 -0.17142857 -0.15714286 -0.14285714 -0.12857143 -0.11428571 -0.1 -0.08571429 -0.07142857 -0.05714286 -0.04285714 -0.02857143 -0.01428571 0 0 0 0 0 0
  line L7 (-20.1149, 3.2402) -> (-20.1771, 3.0947)
  arc A15 (-20.4285, 2.985) -> (-20.1771, 3.0947) centre (-20.361, 3.1733) ccw
  arc A16 (-20.4285, 2.985) -> (-20.6123, 3.0447) centre (-21.5, 0) ccw
  arc A17 (-20.7513, 3.2812) -> (-20.6123, 3.0447) centre (-20.5563, 3.2367) ccw
  line L8 (-20.7513, 3.2812) -> (-20.7161, 3.4355)
  spline S8 degree 5 poles (-20.7161, 3.4355) (-20.7156, 3.4376) (-20.7147, 3.4417) (-20.7136, 3.4479) (-20.7124, 3.4563) (-20.7114, 3.4668) (-20.7107, 3.4774) (-20.7103, 3.4881) (-20.71, 3.4987) (-20.7097, 3.5094) (-20.7096, 3.5201) (-20.7095, 3.5308) (-20.7096, 3.5416) (-20.7098, 3.5524) (-20.7102, 3.5632) (-20.7108, 3.574) (-20.7115, 3.5849) (-20.7124, 3.5957) (-20.7133, 3.6066) (-20.7143, 3.6175) (-20.7154, 3.6285) (-20.7166, 3.6394) (-20.7179, 3.6504) (-20.7194, 3.6613) (-20.7209, 3.6723) (-20.7225, 3.6833) (-20.7243, 3.6943) (-20.7261, 3.7053) (-20.728, 3.7164) (-20.73, 3.7274) (-20.7321, 3.7384) (-20.7343, 3.7495) (-20.7366, 3.7606) (-20.7389, 3.7717) (-20.7414, 3.7827) (-20.7439, 3.7938) (-20.7466, 3.8049) (-20.7493, 3.816) (-20.7521, 3.8272) (-20.7549, 3.8383) (-20.7579, 3.8494) (-20.7609, 3.8605) (-20.7641, 3.8717) (-20.7673, 3.8828) (-20.7705, 3.894) (-20.7739, 3.9051) (-20.7773, 3.9163) (-20.7809, 3.9274) (-20.7845, 3.9386) (-20.7881, 3.9498) (-20.7919, 3.9609) (-20.7957, 3.9721) (-20.7996, 3.9833) (-20.8036, 3.9944) (-20.8076, 4.0056) (-20.8117, 4.0168) (-20.8159, 4.0279) (-20.8202, 4.0391) (-20.8246, 4.0503) (-20.829, 4.0614) (-20.8335, 4.0726) (-20.838, 4.0838) (-20.8427, 4.0949) (-20.8474, 4.1061) (-20.8521, 4.1173) (-20.857, 4.1284) (-20.8619, 4.1396) (-20.8669, 4.1507) (-20.872, 4.1619) (-20.8771, 4.173) (-20.8823, 4.1842) (-20.8865, 4.1931) (-20.8897, 4.1997) (-20.8919, 4.2042) (-20.8929, 4.2064) knots 0 0 0 0 0 0 0.01428571 0.02857143 0.04285714 0.05714286 0.07142857 0.08571429 0.1 0.11428571 0.12857143 0.14285714 0.15714286 0.17142857 0.18571429 0.2 0.21428571 0.22857143 0.24285714 0.25714286 0.27142857 0.28571429 0.3 0.31428571 0.32857143 0.34285714 0.35714286 0.37142857 0.38571429 0.4 0.41428571 0.42857143 0.44285714 0.45714286 0.47142857 0.48571429 0.5 0.51428571 0.52857143 0.54285714 0.55714286 0.57142857 0.58571429 0.6 0.61428571 0.62857143 0.64285714 0.65714286 0.67142857 0.68571429 0.7 0.71428571 0.72857143 0.74285714 0.75714286 0.77142857 0.78571429 0.8 0.81428571 0.82857143 0.84285714 0.85714286 0.87142857 0.88571429 0.9 0.91428571 0.92857143 0.94285714 0.95714286 0.97142857 0.98571429 1 1 1 1 1 1
  arc A18 (-20.8929, 4.2064) -> (-21.2192, 4.2407) centre (-21.5, 0) ccw
  spline S9 degree 5 poles (-21.2192, 4.2407) (-21.2208, 4.2388) (-21.2238, 4.2349) (-21.2283, 4.229) (-21.2343, 4.2211) (-21.2417, 4.2113) (-21.249, 4.2015) (-21.2563, 4.1916) (-21.2635, 4.1818) (-21.2706, 4.1719) (-21.2777, 4.162) (-21.2847, 4.1521) (-21.2916, 4.1421) (-21.2984, 4.1322) (-21.3052, 4.1222) (-21.3119, 4.1122) (-21.3186, 4.1022) (-21.3252, 4.0922) (-21.3317, 4.0821) (-21.3381, 4.0721) (-21.3444, 4.062) (-21.3507, 4.0519) (-21.3569, 4.0418) (-21.3631, 4.0317) (-21.3691, 4.0216) (-21.3751, 4.0115) (-21.381, 4.0013) (-21.3869, 3.9911) (-21.3926, 3.9809) (-21.3983, 3.9708) (-21.4039, 3.9605) (-21.4094, 3.9503) (-21.4149, 3.9401) (-21.4203, 3.9298) (-21.4255, 3.9196) (-21.4307, 3.9093) (-21.4359, 3.899) (-21.4409, 3.8887) (-21.4459, 3.8784) (-21.4508, 3.8681) (-21.4555, 3.8578) (-21.4603, 3.8475) (-21.4649, 3.8371) (-21.4694, 3.8268) (-21.4738, 3.8164) (-21.4782, 3.806) (-21.4824, 3.7956) (-21.4866, 3.7853) (-21.4907, 3.7749) (-21.4947, 3.7645) (-21.4986, 3.754) (-21.5023, 3.7436) (-21.506, 3.7332) (-21.5096, 3.7227) (-21.513, 3.7123) (-21.5164, 3.7018) (-21.5197, 3.6914) (-21.5228, 3.6809) (-21.5259, 3.6705) (-21.5289, 3.66) (-21.5317, 3.6495) (-21.5343, 3.639) (-21.5368, 3.6285) (-21.5391, 3.618) (-21.5413, 3.6075) (-21.5434, 3.597) (-21.5453, 3.5865) (-21.5472, 3.576) (-21.549, 3.5655) (-21.5506, 3.555) (-21.5518, 3.5445) (-21.5524, 3.5361) (-21.5526, 3.5298) (-21.5526, 3.5256) (-21.5525, 3.5235) knots -1 -1 -1 -1 -1 -1 -0.98571429 -0.97142857 -0.95714286 -0.94285714 -0.92857143 -0.91428571 -0.9 -0.88571429 -0.87142857 -0.85714286 -0.84285714 -0.82857143 -0.81428571 -0.8 -0.78571429 -0.77142857 -0.75714286 -0.74285714 -0.72857143 -0.71428571 -0.7 -0.68571429 -0.67142857 -0.65714286 -0.64285714 -0.62857143 -0.61428571 -0.6 -0.58571429 -0.57142857 -0.55714286 -0.54285714 -0.52857143 -0.51428571 -0.5 -0.48571429 -0.47142857 -0.45714286 -0.44285714 -0.42857143 -0.41428571 -0.4 -0.38571429 -0.37142857 -0.35714286 -0.34285714 -0.32857143 -0.31428571 -0.3 -0.28571429 -0.27142857 -0.25714286 -0.24285714 -0.22857143 -0.21428571 -0.2 -0.18571429 -0.17142857 -0.15714286 -0.14285714 -0.12857143 -0.11428571 -0.1 -0.08571429 -0.07142857 -0.05714286 -0.04285714 -0.02857143 -0.01428571 0 0 0 0 0 0
  line L9 (-21.5525, 3.5235) -> (-21.5502, 3.3652)
  arc A19 (-21.7353, 3.1628) -> (-21.5502, 3.3652) centre (-21.7501, 3.3622) ccw
  arc A20 (-21.7353, 3.1628) -> (-21.9274, 3.1426) centre (-21.5, 0) ccw
  arc A21 (-22.1506, 3.3021) -> (-21.9274, 3.1426) centre (-21.9544, 3.3407) ccw
  line L10 (-22.1506, 3.3021) -> (-22.1812, 3.4574)
  spline S10 degree 5 poles (-22.1812, 3.4574) (-22.1816, 3.4595) (-22.1825, 3.4636) (-22.184, 3.4697) (-22.1863, 3.4778) (-22.1897, 3.4879) (-22.1934, 3.4978) (-22.1973, 3.5077) (-22.2013, 3.5176) (-22.2055, 3.5274) (-22.2097, 3.5373) (-22.214, 3.5471) (-22.2184, 3.5569) (-22.223, 3.5666) (-22.2278, 3.5763) (-22.2327, 3.586) (-22.2378, 3.5956) (-22.243, 3.6052) (-22.2482, 3.6148) (-22.2536, 3.6244) (-22.2591, 3.6339) (-22.2646, 3.6434) (-22.2703, 3.6529) (-22.276, 3.6623) (-22.2819, 3.6717) (-22.2879, 3.6811) (-22.2939, 3.6904) (-22.3001, 3.6998) (-22.3063, 3.7091) (-22.3127, 3.7183) (-22.3191, 3.7276) (-22.3256, 3.7368) (-22.3321, 3.746) (-22.3388, 3.7551) (-22.3456, 3.7643) (-22.3524, 3.7734) (-22.3593, 3.7824) (-22.3663, 3.7915) (-22.3734, 3.8005) (-22.3805, 3.8095) (-22.3878, 3.8185) (-22.3951, 3.8274) (-22.4024, 3.8363) (-22.4099, 3.8452) (-22.4174, 3.854) (-22.425, 3.8628) (-22.4327, 3.8716) (-22.4405, 3.8804) (-22.4483, 3.8891) (-22.4562, 3.8978) (-22.4641, 3.9065) (-22.4722, 3.9152) (-22.4803, 3.9238) (-22.4885, 3.9324) (-22.4967, 3.9409) (-22.505, 3.9494) (-22.5134, 3.9579) (-22.5218, 3.9664) (-22.5303, 3.9748) (-22.5389, 3.9832) (-22.5476, 3.9916) (-22.5563, 4) (-22.5651, 4.0083) (-22.5739, 4.0166) (-22.5828, 4.0248) (-22.5918, 4.033) (-22.6008, 4.0412) (-22.6099, 4.0494) (-22.619, 4.0575) (-22.6283, 4.0656) (-22.6376, 4.0737) (-22.645, 4.0801) (-22.6507, 4.0849) (-22.6544, 4.0881) (-22.6563, 4.0897) knots 0 0 0 0 0 0 0.01428571 0.02857143 0.04285714 0.05714286 0.07142857 0.08571429 0.1 0.11428571 0.12857143 0.14285714 0.15714286 0.17142857 0.18571429 0.2 0.21428571 0.22857143 0.24285714 0.25714286 0.27142857 0.28571429 0.3 0.31428571 0.32857143 0.34285714 0.35714286 0.37142857 0.38571429 0.4 0.41428571 0.42857143 0.44285714 0.45714286 0.47142857 0.48571429 0.5 0.51428571 0.52857143 0.54285714 0.55714286 0.57142857 0.58571429 0.6 0.61428571 0.62857143 0.64285714 0.65714286 0.67142857 0.68571429 0.7 0.71428571 0.72857143 0.74285714 0.75714286 0.77142857 0.78571429 0.8 0.81428571 0.82857143 0.84285714 0.85714286 0.87142857 0.88571429 0.9 0.91428571 0.92857143 0.94285714 0.95714286 0.97142857 0.98571429 1 1 1 1 1 1
  arc A22 (-22.6563, 4.0897) -> (-22.9684, 3.9883) centre (-21.5, 0) ccw
  spline S11 degree 5 poles (-22.9684, 3.9883) (-22.969, 3.9859) (-22.9701, 3.9811) (-22.9719, 3.9739) (-22.9741, 3.9643) (-22.9769, 3.9523) (-22.9796, 3.9403) (-22.9822, 3.9284) (-22.9848, 3.9164) (-22.9873, 3.9045) (-22.9897, 3.8926) (-22.9921, 3.8807) (-22.9944, 3.8688) (-22.9966, 3.8569) (-22.9987, 3.845) (-23.0008, 3.8332) (-23.0028, 3.8213) (-23.0047, 3.8095) (-23.0066, 3.7977) (-23.0084, 3.7859) (-23.0101, 3.7741) (-23.0117, 3.7623) (-23.0133, 3.7506) (-23.0148, 3.7389) (-23.0162, 3.7271) (-23.0175, 3.7154) (-23.0188, 3.7038) (-23.02, 3.6921) (-23.0211, 3.6804) (-23.0222, 3.6688) (-23.0231, 3.6572) (-23.024, 3.6456) (-23.0248, 3.6341) (-23.0256, 3.6225) (-23.0262, 3.611) (-23.0268, 3.5995) (-23.0273, 3.588) (-23.0277, 3.5766) (-23.0281, 3.5651) (-23.0283, 3.5537) (-23.0285, 3.5424) (-23.0286, 3.531) (-23.0286, 3.5197) (-23.0285, 3.5084) (-23.0284, 3.4971) (-23.0281, 3.4859) (-23.0278, 3.4746) (-23.0274, 3.4635) (-23.0269, 3.4523) (-23.0263, 3.4412) (-23.0256, 3.4301) (-23.0248, 3.419) (-23.0239, 3.408) (-23.0229, 3.397) (-23.0218, 3.386) (-23.0207, 3.3751) (-23.0194, 3.3643) (-23.018, 3.3534) (-23.0166, 3.3426) (-23.015, 3.3318) (-23.0133, 3.3211) (-23.0115, 3.3105) (-23.0095, 3.2999) (-23.0073, 3.2893) (-23.005, 3.2788) (-23.0026, 3.2684) (-23.0002, 3.258) (-22.9976, 3.2476) (-22.995, 3.2373) (-22.9922, 3.2271) (-22.989, 3.217) (-22.9861, 3.2091) (-22.9837, 3.2032) (-22.982, 3.1994) (-22.9811, 3.1975) knots -1 -1 -1 -1 -1 -1 -0.98571429 -0.97142857 -0.95714286 -0.94285714 -0.92857143 -0.91428571 -0.9 -0.88571429 -0.87142857 -0.85714286 -0.84285714 -0.82857143 -0.81428571 -0.8 -0.78571429 -0.77142857 -0.75714286 -0.74285714 -0.72857143 -0.71428571 -0.7 -0.68571429 -0.67142857 -0.65714286 -0.64285714 -0.62857143 -0.61428571 -0.6 -0.58571429 -0.57142857 -0.55714286 -0.54285714 -0.52857143 -0.51428571 -0.5 -0.48571429 -0.47142857 -0.45714286 -0.44285714 -0.42857143 -0.41428571 -0.4 -0.38571429 -0.37142857 -0.35714286 -0.34285714 -0.32857143 -0.31428571 -0.3 -0.28571429 -0.27142857 -0.25714286 -0.24285714 -0.22857143 -0.21428571 -0.2 -0.18571429 -0.17142857 -0.15714286 -0.14285714 -0.12857143 -0.11428571 -0.1 -0.08571429 -0.07142857 -0.05714286 -0.04285714 -0.02857143 -0.01428571 0 0 0 0 0 0
  line L11 (-22.9811, 3.1975) -> (-22.9146, 3.0539)
  arc A23 (-23.0014, 2.7936) -> (-22.9146, 3.0539) centre (-23.096, 2.9698) ccw
  arc A24 (-23.0014, 2.7936) -> (-23.1687, 2.697) centre (-21.5, 0) ccw
  arc A25 (-23.4374, 2.752) -> (-23.1687, 2.697) centre (-23.2739, 2.8671) ccw
  line L12 (-23.4374, 2.752) -> (-23.5285, 2.8814)
  spline S12 degree 5 poles (-23.5285, 2.8814) (-23.5298, 2.8831) (-23.5322, 2.8865) (-23.5361, 2.8916) (-23.5415, 2.898) (-23.5487, 2.9058) (-23.5561, 2.9134) (-23.5637, 2.9208) (-23.5714, 2.9282) (-23.5792, 2.9355) (-23.587, 2.9428) (-23.595, 2.95) (-23.603, 2.9572) (-23.6112, 2.9642) (-23.6195, 2.9711) (-23.6279, 2.978) (-23.6365, 2.9847) (-23.6451, 2.9914) (-23.6538, 2.998) (-23.6626, 3.0045) (-23.6715, 3.011) (-23.6804, 3.0174) (-23.6894, 3.0237) (-23.6985, 3.03) (-23.7077, 3.0362) (-23.717, 3.0424) (-23.7263, 3.0485) (-23.7357, 3.0545) (-23.7452, 3.0604) (-23.7548, 3.0663) (-23.7644, 3.0722) (-23.7741, 3.0779) (-23.7838, 3.0836) (-23.7936, 3.0893) (-23.8035, 3.0949) (-23.8135, 3.1004) (-23.8235, 3.1059) (-23.8335, 3.1113) (-23.8437, 3.1167) (-23.8539, 3.122) (-23.8641, 3.1272) (-23.8744, 3.1324) (-23.8848, 3.1376) (-23.8952, 3.1426) (-23.9057, 3.1477) (-23.9162, 3.1526) (-23.9268, 3.1575) (-23.9375, 3.1624) (-23.9482, 3.1672) (-23.9589, 3.1719) (-23.9697, 3.1766) (-23.9806, 3.1812) (-23.9915, 3.1858) (-24.0024, 3.1903) (-24.0134, 3.1948) (-24.0245, 3.1992) (-24.0356, 3.2036) (-24.0468, 3.2079) (-24.058, 3.2121) (-24.0692, 3.2163) (-24.0805, 3.2204) (-24.0919, 3.2245) (-24.1033, 3.2285) (-24.1147, 3.2325) (-24.1262, 3.2364) (-24.1378, 3.2403) (-24.1493, 3.2441) (-24.161, 3.2479) (-24.1726, 3.2516) (-24.1844, 3.2552) (-24.1961, 3.2588) (-24.2056, 3.2616) (-24.2127, 3.2637) (-24.2174, 3.2651) (-24.2198, 3.2658) knots 0 0 0 0 0 0 0.01428571 0.02857143 0.04285714 0.05714286 0.07142857 0.08571429 0.1 0.11428571 0.12857143 0.14285714 0.15714286 0.17142857 0.18571429 0.2 0.21428571 0.22857143 0.24285714 0.25714286 0.27142857 0.28571429 0.3 0.31428571 0.32857143 0.34285714 0.35714286 0.37142857 0.38571429 0.4 0.41428571 0.42857143 0.44285714 0.45714286 0.47142857 0.48571429 0.5 0.51428571 0.52857143 0.54285714 0.55714286 0.57142857 0.58571429 0.6 0.61428571 0.62857143 0.64285714 0.65714286 0.67142857 0.68571429 0.7 0.71428571 0.72857143 0.74285714 0.75714286 0.77142857 0.78571429 0.8 0.81428571 0.82857143 0.84285714 0.85714286 0.87142857 0.88571429 0.9 0.91428571 0.92857143 0.94285714 0.95714286 0.97142857 0.98571429 1 1 1 1 1 1
  arc A26 (-24.2198, 3.2658) -> (-24.4636, 3.0462) centre (-21.5, 0) ccw